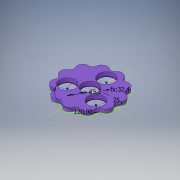
# Autodesk Inventor part: Excenter
Saved by Autodesk Inventor 2018.3 (Build 223284000, 284)
## iProperties
Created: 2018-07-20
Part Number: Excenter
Material: Generisch
Document SubType Name: Modeling
Designer: JochenAlt
Density: 1 g/cm^3
Appearance: Violett
Author: JochenAlt
Autodesk Inventor part; units mm, degrees
ref_plane "YZ Plane" through (0, 0, 0) normal (1, 0, 0) x (0, 1, 0)
ref_plane "XZ Plane" through (0, 0, 0) normal (0, 1, 0) x (-1, 0, 0)
ref_plane "XY Plane" through (0, 0, 0) normal (0, 0, 1) x (1, 0, 0)
sketch "Skizze1" plane through (0, 0, 0) normal (0, 0, 1) x (1, 0, 0)
  line L0 (0, 41.4451) -> (0, -41.4451) construction
  line L1 (-40.8713, 0) -> (41.0136, 0) construction
  circle A0 centre (0, 0) radius 7.6
  line L2 (0, 0) -> (25.1147, -14.5) construction
  line L3 (0, 0) -> (-25.1147, -14.5) construction
  circle A1 centre (14.0296, -8.1) radius 7.6
  circle A2 centre (-14.0296, -8.1) radius 7.6
  circle A3 centre (0, 16.2) radius 7.6
  circle A4 centre (0, 0) radius 16.2 construction
  spline S0 degree 5 poles (25, 0) (24.9981, -0.6158) (25.1441, -1.2181) (25.4052, -1.8106) (25.9558, -2.4315) (26.5188, -3.0385) (26.6567, -3.2055) (26.9569, -3.6146) (27.1965, -4.063) (27.3136, -4.3303) (27.5368, -4.9625) (27.6569, -5.6231) (27.6929, -6.0012) (27.7036, -6.7985) (27.5815, -7.5871) (27.4821, -7.994) (27.2221, -8.7656) (26.837, -9.4827) (26.6212, -9.8149) (26.1822, -10.3792) (25.6582, -10.8639) (25.4086, -11.0624) (24.9552, -11.3653) (24.4636, -11.5987) (24.2529, -11.6819) (23.669, -11.8708) (23.0679, -11.9986) (22.6992, -12.1234) (21.599, -12.6599) (20.7928, -13.6142) (20.4455, -14.4411) (20.4092, -15.5126) (20.606, -16.544) (20.648, -16.7707) (20.7137, -17.261) (20.7122, -17.7565) (20.6919, -18.0202) (20.6002, -18.6365) (20.414, -19.2321) (20.2781, -19.565) (19.9305, -20.2548) (19.4732, -20.8783) (19.2005, -21.19) (18.609, -21.7603) (17.9305, -22.2236) (17.575, -22.4247) (16.8909, -22.7377) (16.1656, -22.9338) (15.8273, -22.9976) (15.2387, -23.0581) (14.6487, -23.029) (14.4029, -22.9996) (13.8989, -22.9032) (13.4119, -22.7422) (13.1627, -22.6526) (12.0646, -22.3284) (10.8877, -22.3671) (9.9934, -22.7395) (9.1021, -23.5611) (8.5702, -24.6124) (8.4603, -24.886) (8.2645, -25.3842) (8.0069, -25.8534) (7.878, -26.0553) (7.5355, -26.5169) (7.1276, -26.923) (6.8703, -27.1392) (6.2695, -27.5705) (5.6052, -27.8981) (5.2281, -28.0454) (4.4419, -28.2787) (3.6277, -28.3773) (3.2117, -28.392) (2.4303, -28.3525) (1.667, -28.1843) (1.3162, -28.0769) (0.7222, -27.8384) (0.1733, -27.5105) (-0.0505, -27.3538) (-0.4347, -27.0399) (-0.7703, -26.6767) (-0.9127, -26.5061) (-1.5176, -25.7303) (-2.2508, -25.0515) (-3.0125, -24.7341) (-4.2592, -24.577) (-5.439, -24.9574) (-5.8516, -25.1607) (-6.3938, -25.565) (-6.9624, -25.9274) (-7.1566, -26.0341) (-7.6363, -26.2598) (-8.145, -26.4143) (-8.4478, -26.48) (-9.1411, -26.5772) (-9.842, -26.5613) (-10.231, -26.5192) (-11.0257, -26.366) (-11.7841, -26.0821) (-12.1628, -25.9021) (-12.8571, -25.4957) (-13.4736, -24.9798) (-13.7482, -24.7087) (-14.1938, -24.1866) (-14.5498, -23.6006) (-14.6864, -23.3328) (-14.8853, -22.853) (-15.0123, -22.3514) (-15.0538, -22.1369) (-15.1464, -21.3964) (-15.219, -20.65) (-15.401, -20.1368) (-16.0101, -19.0446) (-17.042, -18.3232) (-17.7274, -18.0511) (-18.6446, -18.0074) (-19.5517, -18.0512) (-19.7697, -18.05) (-20.2677, -18.0225) (-20.7587, -17.9239) (-21.0306, -17.8479) (-21.6469, -17.6254) (-22.2211, -17.3085) (-22.5316, -17.1008) (-23.1507, -16.6102) (-23.6802, -16.023) (-23.9324, -15.6899) (-24.3686, -14.9982) (-24.683, -14.2436) (-24.8056, -13.862) (-24.9685, -13.1523) (-25.0134, -12.4267) (-25.009, -12.0991) (-24.9545, -11.5418) (-24.8192, -10.9993) (-24.7473, -10.7781) (-24.5379, -10.2502) (-24.2666, -9.7509) (-24.1234, -9.448) (-23.73, -8.3097) (-23.7997, -7.0761) (-24.1571, -6.2007) (-24.9319, -5.3761) (-25.8772, -4.8075) (-26.0893, -4.6873) (-26.5131, -4.4221) (-26.8983, -4.1029) (-27.083, -3.9259) (-27.4906, -3.4762) (-27.8251, -2.9687) (-27.9934, -2.6595) (-28.3043, -1.9635) (-28.4964, -1.2249) (-28.5655, -0.8192) (-28.6345, 0) (-28.5655, 0.8192) (-28.4964, 1.2249) (-28.3043, 1.9635) (-27.9934, 2.6595) (-27.8251, 2.9687) (-27.4906, 3.4762) (-27.083, 3.9259) (-26.8983, 4.1029) (-26.5131, 4.4221) (-26.0893, 4.6873) (-25.8772, 4.8075) (-24.9319, 5.3761) (-24.1571, 6.2007) (-23.7997, 7.0761) (-23.73, 8.3097) (-24.1234, 9.448) (-24.2666, 9.7509) (-24.5379, 10.2502) (-24.7473, 10.7781) (-24.8192, 10.9993) (-24.9545, 11.5418) (-25.009, 12.0991) (-25.0134, 12.4267) (-24.9685, 13.1523) (-24.8056, 13.862) (-24.683, 14.2436) (-24.3686, 14.9982) (-23.9324, 15.6899) (-23.6802, 16.023) (-23.1507, 16.6102) (-22.5316, 17.1008) (-22.2211, 17.3085) (-21.6469, 17.6254) (-21.0306, 17.8479) (-20.7587, 17.9239) (-20.2677, 18.0225) (-19.7697, 18.05) (-19.5517, 18.0512) (-18.6446, 18.0074) (-17.7274, 18.0511) (-17.042, 18.3232) (-16.0101, 19.0446) (-15.401, 20.1368) (-15.219, 20.65) (-15.1464, 21.3964) (-15.0538, 22.1369) (-15.0123, 22.3514) (-14.8853, 22.853) (-14.6864, 23.3328) (-14.5498, 23.6006) (-14.1938, 24.1866) (-13.7482, 24.7087) (-13.4736, 24.9798) (-12.8571, 25.4957) (-12.1628, 25.9021) (-11.7841, 26.0821) (-11.0257, 26.366) (-10.231, 26.5192) (-9.842, 26.5613) (-9.1411, 26.5772) (-8.4478, 26.48) (-8.145, 26.4143) (-7.6363, 26.2598) (-7.1566, 26.0341) (-6.9624, 25.9274) (-6.3938, 25.565) (-5.8516, 25.1607) (-5.439, 24.9574) (-4.2592, 24.577) (-3.0125, 24.7341) (-2.2508, 25.0515) (-1.5176, 25.7303) (-0.9127, 26.5061) (-0.7703, 26.6767) (-0.4347, 27.0399) (-0.0505, 27.3538) (0.1733, 27.5105) (0.7222, 27.8384) (1.3162, 28.0769) (1.667, 28.1843) (2.4303, 28.3525) (3.2117, 28.392) (3.6277, 28.3773) (4.4419, 28.2787) (5.2281, 28.0454) (5.6052, 27.8981) (6.2695, 27.5705) (6.8703, 27.1392) (7.1276, 26.923) (7.5355, 26.5169) (7.878, 26.0553) (8.0069, 25.8534) (8.2645, 25.3842) (8.4603, 24.886) (8.5702, 24.6124) (9.1021, 23.5611) (9.9934, 22.7395) (10.8877, 22.3671) (12.0646, 22.3284) (13.1627, 22.6526) (13.4119, 22.7422) (13.8989, 22.9032) (14.4029, 22.9996) (14.6487, 23.029) (15.2387, 23.0581) (15.8273, 22.9976) (16.1656, 22.9338) (16.8909, 22.7377) (17.575, 22.4247) (17.9305, 22.2236) (18.609, 21.7603) (19.2005, 21.19) (19.4732, 20.8783) (19.9305, 20.2548) (20.2781, 19.565) (20.414, 19.2321) (20.6002, 18.6365) (20.6919, 18.0202) (20.7122, 17.7565) (20.7137, 17.261) (20.648, 16.7707) (20.606, 16.544) (20.4092, 15.5126) (20.4455, 14.4411) (20.7928, 13.6142) (21.599, 12.6599) (22.6992, 12.1234) (23.0679, 11.9986) (23.669, 11.8708) (24.2529, 11.6819) (24.4636, 11.5987) (24.9552, 11.3653) (25.4086, 11.0624) (25.6582, 10.8639) (26.1822, 10.3792) (26.6212, 9.8149) (26.837, 9.4827) (27.2221, 8.7656) (27.4821, 7.994) (27.5815, 7.5871) (27.7036, 6.7985) (27.6929, 6.0012) (27.6569, 5.6231) (27.5368, 4.9625) (27.3136, 4.3303) (27.1965, 4.063) (26.9569, 3.6146) (26.6567, 3.2055) (26.5188, 3.0385) (25.9558, 2.4315) (25.4052, 1.8106) (25.1441, 1.2181) (24.9981, 0.6158) (25, 0) knots 0 0 0 0 0 0 0.015805 0.015805 0.015805 0.021374 0.021374 0.021374 0.028875 0.028875 0.028875 0.038628 0.038628 0.038628 0.049382 0.049382 0.049382 0.059557 0.059557 0.059557 0.06775 0.06775 0.06775 0.073572 0.073572 0.073572 0.083574 0.083574 0.083574 0.104736 0.104736 0.104736 0.110677 0.110677 0.110677 0.11748 0.11748 0.11748 0.126714 0.126714 0.126714 0.137349 0.137349 0.137349 0.147836 0.147836 0.147836 0.156678 0.156678 0.156678 0.163044 0.163044 0.163044 0.169887 0.169887 0.169887 0.192492 0.192492 0.192492 0.200112 0.200112 0.200112 0.206274 0.206274 0.206274 0.214907 0.214907 0.214907 0.225304 0.225304 0.225304 0.235991 0.235991 0.235991 0.24541 0.24541 0.24541 0.252442 0.252442 0.252442 0.258157 0.258157 0.258157 0.277862 0.277862 0.277862 0.289577 0.289577 0.289577 0.295268 0.295268 0.295268 0.303236 0.303236 0.303236 0.313282 0.313282 0.313282 0.324049 0.324049 0.324049 0.333956 0.333956 0.333956 0.341689 0.341689 0.341689 0.347295 0.347295 0.347295 0.360974 0.360974 0.360974 0.378861 0.378861 0.378861 0.384456 0.384456 0.384456 0.391723 0.391723 0.391723 0.401314 0.401314 0.401314 0.412041 0.412041 0.412041 0.422333 0.422333 0.422333 0.430748 0.430748 0.430748 0.436729 0.436729 0.436729 0.445379 0.445379 0.445379 0.467518 0.467518 0.467518 0.473811 0.473811 0.473811 0.480391 0.480391 0.480391 0.489432 0.489432 0.489432 0.5 0.5 0.5 0.510568 0.510568 0.510568 0.519609 0.519609 0.519609 0.526189 0.526189 0.526189 0.532482 0.532482 0.532482 0.554621 0.554621 0.554621 0.563271 0.563271 0.563271 0.569252 0.569252 0.569252 0.577667 0.577667 0.577667 0.587959 0.587959 0.587959 0.598686 0.598686 0.598686 0.608277 0.608277 0.608277 0.615544 0.615544 0.615544 0.621139 0.621139 0.621139 0.639026 0.639026 0.639026 0.652705 0.652705 0.652705 0.658311 0.658311 0.658311 0.666044 0.666044 0.666044 0.675951 0.675951 0.675951 0.686718 0.686718 0.686718 0.696764 0.696764 0.696764 0.704732 0.704732 0.704732 0.710423 0.710423 0.710423 0.722138 0.722138 0.722138 0.741843 0.741843 0.741843 0.747558 0.747558 0.747558 0.75459 0.75459 0.75459 0.764009 0.764009 0.764009 0.774696 0.774696 0.774696 0.785093 0.785093 0.785093 0.793726 0.793726 0.793726 0.799888 0.799888 0.799888 0.807508 0.807508 0.807508 0.830113 0.830113 0.830113 0.836956 0.836956 0.836956 0.843322 0.843322 0.843322 0.852164 0.852164 0.852164 0.862651 0.862651 0.862651 0.873286 0.873286 0.873286 0.88252 0.88252 0.88252 0.889323 0.889323 0.889323 0.895264 0.895264 0.895264 0.916426 0.916426 0.916426 0.926428 0.926428 0.926428 0.93225 0.93225 0.93225 0.940443 0.940443 0.940443 0.950618 0.950618 0.950618 0.961372 0.961372 0.961372 0.971125 0.971125 0.971125 0.978626 0.978626 0.978626 0.984195 0.984195 0.984195 1 1 1 1 1 1
  circle A5 centre (0, 0) radius 25 construction
  dimension "d1" = 15.2
  dimension "d2" = 120
  dimension "d3" = 32.4
  dimension "d12" = 25
  constraints: 5 centre point, 4 end point, 4 point on line, 3 equal radius, 3 point on circle, 2 coincident, 1 horizontal alignment, 5 other
  measures "d1" diameter of A0
  measures "d2" angle of L2 L3
  measures "d3" diameter of A4
  measures "d12" distance of point (25, 0) L2.start
extrude "Extrusion1" add sketch "Skizze1" along normal blind 4
equation "curve S0 of \"Skizze1\": x = (29.9*cos(t))-(3,1*cos(t+atan(sin(-11*t)/((29,9/1.8/12)-cos(-11*t)))))-(1.8*cos(12*t)); y = (-29.9*sin(t))+(3,1*sin(t+atan(sin(-11*t)/((29.9/1.8/12)-cos(-11*t)))))+(1.8*sin("
